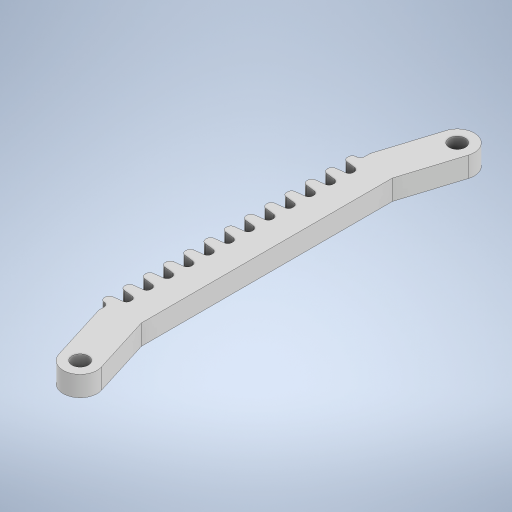
# Autodesk Inventor part: Direcciondeopalaaa
Saved by Autodesk Inventor 2023 (Build 270158000, 158)
## iProperties
Created: 2025-03-18
Part Number: Direcciondeopalaaa
Material: Genérico
Document SubType Name: Modeling
Designer: angel.dasilva
Density: 1 g/cm^3
Appearance: Valor por defecto
Author: angel.dasilva
Autodesk Inventor part; units mm, degrees
ref_plane "YZ Plane" through (0, 0, 0) normal (1, 0, 0) x (0, 1, 0)
ref_plane "XZ Plane" through (0, 0, 0) normal (0, 1, 0) x (-1, 0, 0)
ref_plane "XY Plane" through (0, 0, 0) normal (0, 0, 1) x (1, 0, 0)
sketch "Boceto1" plane through (0, 0, 0) normal (0, 1, 0) x (-1, 0, 0)
  line L0 (0, -67) -> (-8, -64.5)
  line L1 (-8, -2.5) -> (0, 0)
  line L2 (-8, -64.5) -> (-12.4741, -78.8172)
  line L3 (0, -67) -> (-4.4741, -81.3172)
  circle A0 centre (-8.4741, -80.0672) radius 2
  arc A1 (-12.4741, -78.8172) -> (-4.4741, -81.3172) centre (-8.4741, -80.0672) ccw
  line L4 (0, 0) -> (-8, -2.5)
  line L5 (-8, -2.5) -> (-12.4741, 11.8172)
  line L6 (0, 0) -> (-4.4741, 14.3172)
  circle A2 centre (-8.4741, 13.0672) radius 2
  arc A3 (-4.4741, 14.3172) -> (-12.4741, 11.8172) centre (-8.4741, 13.0672) ccw
  line L7 (-2, -65) -> (-2, -3)
  line L8 (0, -67) -> (0, -65)
  line L9 (-8, -64.5) -> (-8, -2.5)
  line L10 (-2, -65) -> (-2, -64.5)
  line L11 (-2, -64.5) -> (-2, -63.5)
  line L12 (2, -63.5) -> (2, -64.5)
  line L13 (2, -64.5) -> (-2, -65)
  line L14 (2, -63.5) -> (2, -62.5)
  line L15 (2, -62.5) -> (-2, -62)
  line L16 (-2, -62) -> (-2, -60)
  line L17 (-2, -60) -> (-2, -58.5)
  line L18 (2, -59.5) -> (-2, -60)
  line L19 (2, -58.5) -> (2, -59.5)
  line L20 (2, -58.5) -> (2, -57.5)
  line L21 (2, -57.5) -> (-2, -57)
  line L22 (2, -54.5) -> (-2, -55)
  line L23 (2, -53.5) -> (2, -54.5)
  line L24 (2, -53.5) -> (2, -52.5)
  line L25 (2, -52.5) -> (-2, -52)
  line L26 (2, -49.5) -> (-2, -50)
  line L27 (2, -48.5) -> (2, -49.5)
  line L28 (2, -48.5) -> (2, -47.5)
  line L29 (2, -47.5) -> (-2, -47)
  line L30 (2, -44.5) -> (-2, -45)
  line L31 (2, -43.5) -> (2, -44.5)
  line L32 (2, -43.5) -> (2, -42.5)
  line L33 (2, -42.5) -> (-2, -42)
  line L34 (2, -39.5) -> (-2, -40)
  line L35 (2, -38.5) -> (2, -39.5)
  line L36 (2, -38.5) -> (2, -37.5)
  line L37 (2, -37.5) -> (-2, -37)
  line L38 (2, -34.5) -> (-2, -35)
  line L39 (2, -33.5) -> (2, -34.5)
  line L40 (2, -33.5) -> (2, -32.5)
  line L41 (2, -32.5) -> (-2, -32)
  line L42 (2, -29.5) -> (-2, -30)
  line L43 (2, -28.5) -> (2, -29.5)
  line L44 (2, -28.5) -> (2, -27.5)
  line L45 (2, -27.5) -> (-2, -27)
  line L46 (2, -24.5) -> (-2, -25)
  line L47 (2, -23.5) -> (2, -24.5)
  line L48 (2, -23.5) -> (2, -22.5)
  line L49 (2, -22.5) -> (-2, -22)
  line L50 (2, -19.5) -> (-2, -20)
  line L51 (2, -18.5) -> (2, -19.5)
  line L52 (2, -18.5) -> (2, -17.5)
  line L53 (2, -17.5) -> (-2, -17)
  line L54 (2, -14.5) -> (-2, -15)
  line L55 (2, -13.5) -> (2, -14.5)
  line L56 (2, -13.5) -> (2, -12.5)
  line L57 (2, -12.5) -> (-2, -12)
  line L58 (2, -9.5) -> (-2, -10)
  line L59 (2, -8.5) -> (2, -9.5)
  line L60 (2, -8.5) -> (2, -7.5)
  line L61 (2, -7.5) -> (-2, -7)
  line L62 (2, -4.5) -> (-2, -5)
  line L63 (2, -3.5) -> (2, -4.5)
  line L64 (2, -3.5) -> (2, -2.5)
  line L65 (2, -2.5) -> (-2, -2)
  line L66 (-2, -2) -> (-2, -3)
  line L67 (0, 0) -> (0, -2.25)
  line L68 (0, -65) -> (0, -64.75)
  point P0 (0, -65)
  point P1 (-2, -62)
  point P2 (-2, -57)
  point P3 (-2, -55)
  point P4 (-2, -52)
  point P5 (-2, -50)
  point P6 (-2, -47)
  point P7 (-2, -45)
  point P8 (-2, -42)
  point P9 (-2, -40)
  point P10 (-2, -37)
  point P11 (-2, -35)
  point P12 (-2, -32)
  point P13 (-2, -30)
  point P14 (-2, -27)
  point P15 (-2, -25)
  point P16 (-2, -22)
  point P17 (-2, -10)
  point P18 (-2, -7)
  point P19 (-2, -5)
  dimension "d0" = 67
  dimension "d6" = 4
  dimension "d20" = 2
  dimension "d22" = 0.5
  dimension "d23" = 1
  dimension "d25" = 1
  dimension "d27" = 2
  dimension "d28" = 1.5
  dimension "d32" = 5
  constraints: 136 end point, 60 vertical alignment, 24 collinear, 24 parallel, 4 centre point, 4 point on circle, 2 coincident, 2 midpoint, 2 vertical, 8 other
  measures "d0" distance of L0.start L1.end
  measures "d6" diameter of A0
  measures "d20" distance of L0.start L8.end
  measures "d22" distance of L10.start L10.end
  measures "d23" distance of L10.end L11.end
  measures "d25" distance of L12.start L12.end
  measures "d27" distance of L15.end L16.end
  measures "d28" distance of L16.end L17.end
  measures "d32" distance of L12.end L18.start
extrude "Extrusión1" add sketch "Boceto1" along normal blind 5
fillet "Empalme1" radius 1 54 edges at (0, 2.5, 0) (0, 2.5, -2.25) (-2, 2.5, -2.5) (-2, 2.5, -4.5) (2, 2.5, -5) (-2, 2.5, -7.5) (2, 2.5, -7) (2, 2.5, -10) (-2, 2.5, -9.5) (-2, 2.5, -12.5) (-2, 2.5, -14.5) (2, 2.5, -12) (2, 2.5, -15) (2, 2.5, -17) (-2, 2.5, -17.5) (-2, 2.5, -19.5) (2, 2.5, -20) (2, 2.5, -22) (-2, 2.5, -22.5) (-2, 2.5, -24.5) (2, 2.5, -25) (2, 2.5, -27) (-2, 2.5, -27.5) (-2, 2.5, -29.5) (2, 2.5, -30) (2, 2.5, -35) (2, 2.5, -32) (-2, 2.5, -32.5) (-2, 2.5, -34.5) (2, 2.5, -37) (-2, 2.5, -37.5) (-2, 2.5, -39.5) (2, 2.5, -40) (2, 2.5, -42) (-2, 2.5, -42.5) (-2, 2.5, -44.5) (2, 2.5, -45) (2, 2.5, -47) (-2, 2.5, -47.5) (-2, 2.5, -49.5) (2, 2.5, -50) (2, 2.5, -52) (-2, 2.5, -52.5) (-2, 2.5, -54.5) (2, 2.5, -55) (2, 2.5, -57) (-2, 2.5, -57.5) (-2, 2.5, -59.5) (2, 2.5, -60) (2, 2.5, -62) (-2, 2.5, -62.5) (-2, 2.5, -64.5) (0, 2.5, -67) (0, 2.5, -64.75)
